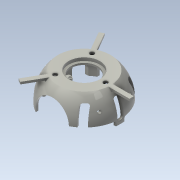
# Autodesk Inventor part: RobotHoedje
Saved by Autodesk Inventor 2020.3 (Build 243373000, 373)
## iProperties
Created: 2020-10-22
Part Number: RobotHoedje
Material: Acetal Resin, Black
Document SubType Name: Modeling
Designer: Britt
Density: 1.425 g/cm^3
Appearance: Smooth - Ivory
Author: Britt
Autodesk Inventor part; units mm, degrees
ref_plane "YZ Plane" through (0, 0, 0) normal (1, 0, 0) x (0, 1, 0)
ref_plane "XZ Plane" through (0, 0, 0) normal (0, 1, 0) x (-1, 0, 0)
ref_plane "XY Plane" through (0, 0, 0) normal (0, 0, 1) x (1, 0, 0)
sketch "Sketch1" plane through (0, 0, 0) normal (0, 1, 0) x (-1, 0, 0)
  circle A0 centre (0, 0) radius 81.5
  line L0 (0, 81.5) -> (0, 79.5)
  line L1 (0, 79.5) -> (17.9444, 79.5)
  line L2 (0, 79.5) -> (-17.9444, 79.5)
  dimension "d0" = 163
  dimension "d13" = 2
  constraints: 6 end point, 3 point on circle, 1 centre point, 1 coincident, 1 perpendicular, 1 point on line, 1 vertical
  measures "d0" diameter of A0
  measures "d13" distance of L0.start L0.end
extrude "Extrusion1" add sketch "Sketch1" along normal blind 90 contours A0 L2 L1
fillet "Fillet1" radius 80 1 edges at (0, 90, -81.5)
shell "Shell1" thickness 5 removed faces 1 at (-16.0199, 0, 6.9823)
sketch "Sketch3" plane through (-17.9444, 0, 79.5) normal (0, 0, 1) x (1, 0, 0)
  line L0 (17.9444, 0) -> (17.9444, 10)
  circle A0 centre (17.9444, 10) radius 37.5
  line L1 (-19.5556, 10) -> (-19.5556, 0)
  line L2 (55.4444, 10) -> (55.4444, 0)
  line L3 (99.4444, 0) -> (-63.5556, 0) projected
  line L4 (55.4444, 0) -> (-19.5556, 0)
  line L5 (0, 0) -> (35.8887, 0) projected
  dimension "d14" = 10
  dimension "d15" = 75
  constraints: 8 end point, 3 vertical, 2 point on circle, 1 centre point, 1 coincident, 1 collinear, 1 point on line, 1 tangent
  measures "d14" distance of L0.start L0.end
  measures "d15" diameter of A0
extrude "Extrusion3" cut sketch "Sketch3" against normal through all both and the other way through all contours A0 L3 | L2 L3 A0 | A0 L3 L1 picked at (4.1693, 13.1062)
sketch "Sketch5" plane through (0, 90, 0) normal (0, 1, 0) x (1, 0, 0)
  circle A0 centre (0, 0) radius 1.5 projected
  circle A1 centre (0, 0) radius 35.5
  dimension "d24" = 71
  constraints: 1 centre point, 1 coincident
  measures "d24" diameter of A1
extrude "Extrusion5" cut sketch "Sketch5" against normal through all
ref_plane "Work Plane3" through (0, 78, 0) normal (0, 1, 0) x (1, 0, 0)
sketch "Sketch6" plane through (0, 78, 0) normal (0, 1, 0) x (1, 0, 0)
  line L0 (-10, -40.5) -> (10, -40.5)
  circle A0 centre (0, 0) radius 35.5 projected
  line L1 (10, -30.5) -> (-10, -40.5) construction
  line L2 (-10, -30.5) -> (10, -40.5) construction
  line L3 (10, 40.5) -> (-10, 40.5)
  line L4 (10, 40.5) -> (-10, 30.5) construction
  line L5 (-10, 40.5) -> (10, 30.5) construction
  line L6 (-40.5, -10) -> (-40.5, 10)
  line L7 (-30.5, -10) -> (-40.5, 10) construction
  line L8 (-40.5, -10) -> (-30.5, 10) construction
  line L9 (40.5, 10) -> (40.5, -10)
  line L10 (30.5, 10) -> (40.5, -10) construction
  line L11 (40.5, 10) -> (30.5, -10) construction
  circle A1 centre (0, 0) radius 40.5
  point P0 (0, -35.5)
  point P1 (0, 35.5)
  point P2 (-35.5, 0)
  point P3 (35.5, 0)
  dimension "d28" = 20
  dimension "d29" = 10
  dimension "d30" = 20
  dimension "d31" = 10
  dimension "d32" = 10
  dimension "d33" = 20
  dimension "d34" = 10
  dimension "d35" = 20
  constraints: 24 end point, 8 midpoint, 4 point on circle, 1 centre point, 1 coincident, 1 horizontal
  measures "d28" distance of L0.end L0.start
  measures "d29" distance of L2.start L0.start
  measures "d30" distance of L5.end L4.end
  measures "d31" distance of L4.end L3.end
  measures "d32" distance of L6.end L8.end
  measures "d33" distance of L6.start L6.end
  measures "d34" distance of L9.end L11.end
  measures "d35" distance of L9.start L9.end
extrude "Extrusion6" add sketch "Sketch6" against normal blind 20
sketch "Sketch7" plane through (0, 58, 0) normal (0, -1, 0) x (1, 0, 0)
  circle A0 centre (0, 0) radius 1.5 projected
  circle A1 centre (0, 0) radius 38.5714
  circle A2 centre (0, 0) radius 30
  dimension "d38" = 60
  constraints: 2 centre point, 2 coincident
  measures "d38" diameter of A2
extrude "Extrusion7" add sketch "Sketch7" along normal blind 4 contours A1
sketch "Sketch8" plane through (0, 0, 0) normal (0, -1, 0) x (1, 0, 0)
  arc A0 (76.2643, 6) -> (38.7342, 65.969) centre (0, 0) ccw projected
  line L0 (61.5, 6) -> (76.2643, 6) projected
  line L1 (76.097, 6) -> (81.2788, 6)
  arc A1 (41.2658, -70.2807) -> (41.2658, 70.2807) centre (0, 0) ccw projected
  line L2 (76.2643, -6) -> (61.5, -6) projected
  line L3 (76.097, -6) -> (81.2788, -6)
  line L4 (39.2915, 69.117) -> (34.9018, 73.1705)
  line L5 (34.9018, 73.1705) -> (33.5102, 67.8706)
  line L6 (33.5102, 67.8706) -> (38.7342, 65.969)
  line L7 (41.2658, -70.2807) -> (36.538, -72.9193)
  line L8 (36.538, -72.9193) -> (34.4671, -67.6441)
  arc A2 (38.7342, -65.969) -> (76.2643, -6) centre (0, 0) ccw projected
  line L9 (34.4671, -67.6441) -> (38.7342, -65.969)
  line L10 (76.097, 6) -> (61.5, 6)
  line L11 (33.5102, 67.8706) -> (61.5, 6)
  line L12 (61.5, -6) -> (34.4671, -67.6441)
  line L13 (81.2788, -6) -> (84.4133, -6)
  line L14 (84.4133, -6) -> (69.6893, -61.2083)
  line L15 (69.6893, -61.2083) -> (36.538, -72.9193)
  line L16 (81.2788, 6) -> (84.4133, 6)
  line L17 (84.4133, 6) -> (69.5528, 69.3789)
  line L18 (69.5528, 69.3789) -> (34.9018, 73.1705)
  line L19 (76.097, 6) -> (75.9085, 9.4949)
  arc A3 (-37.5, 66.6783) -> (-37.5, -66.6783) centre (0, 0) ccw projected
  line L20 (75.9085, 9.4949) -> (83.5938, 9.4949)
  line L21 (75.9085, 9.4949) -> (59.9189, 9.4949)
  line L22 (76.097, -6) -> (75.9085, -9.4949)
  line L23 (75.9085, -9.4949) -> (83.4812, -9.4949)
  line L24 (75.9085, -9.4949) -> (59.8849, -9.4949)
  point P0 (41.2658, 70.0874)
  point P1 (41.2658, 70.2807)
  point P2 (59.9674, -9.4949)
  dimension "d153" = 3.5
  dimension "d154" = 3.5
  constraints: 46 end point, 6 point on line, 4 horizontal, 3 point on circle, 1 collinear, 1 parallel, 1 perpendicular
  measures "d153" distance of L1.start L19.end
  measures "d154" distance of L3.start L22.end
extrude "Extrusion23" cut sketch "Sketch8" against normal blind 10 contours L21 L11 L6 A0 | A0 L6 L5 L18 L17 L20 | L7 L8 L9 A2 L23 A1 | A1 L23 L14 L15 L7 | A2 L9 L12 L24
sketch "Sketch9" plane through (0, 85, 0) normal (0, -1, 0) x (1, 0, 0)
  circle A0 centre (0, 0) radius 38.5714 projected
  line L0 (0, 38.5714) -> (-15, 38.5714)
  line L1 (-15, 38.5714) -> (-15, 68.5714)
  line L2 (-15, 68.5714) -> (0, 68.5714)
  line L3 (0, 68.5714) -> (0, 38.5714)
  line L4 (0, 38.5714) -> (15, 38.5714)
  line L5 (15, 38.5714) -> (15, 68.5714)
  line L6 (15, 68.5714) -> (0, 68.5714)
  line L7 (0, 68.5714) -> (0, 38.5714)
  arc A1 (-40.5, 0) -> (-40.5, 0) centre (0, 0) ccw projected
  line L8 (0, -40.5) -> (-15, -40.5)
  line L9 (-15, -40.5) -> (-15, -70.5)
  line L10 (-15, -70.5) -> (0, -70.5)
  line L11 (0, -70.5) -> (0, -40.5)
  line L12 (0, -70.5) -> (15, -70.5)
  line L13 (15, -70.5) -> (15, -40.5)
  line L14 (15, -40.5) -> (0, -40.5)
  line L15 (0, -40.5) -> (0, -70.5)
  arc A2 (-40.5, 0) -> (-40.5, 0) centre (0, 0) ccw projected
  line L16 (40.5, 0) -> (70.5, 0)
  line L17 (70.5, 0) -> (70.5, 15)
  line L18 (70.5, 15) -> (40.5, 15)
  line L19 (40.5, 15) -> (40.5, 0)
  line L20 (70.5, 0) -> (40.5, 0)
  line L21 (40.5, 0) -> (40.5, -15)
  line L22 (40.5, -15) -> (70.5, -15)
  line L23 (70.5, -15) -> (70.5, 0)
  point P0 (0, 68.5714)
  dimension "d43" = 15
  dimension "d44" = 30
  dimension "d45" = 15
  dimension "d46" = 30
  dimension "d47" = 30
  dimension "d48" = 15
  dimension "d49" = 15
  constraints: 48 end point, 12 parallel, 6 horizontal, 6 perpendicular, 6 point on line, 2 point on circle, 2 other
  measures "d43" distance of L1.end L2.end
  measures "d44" distance of L0.end L1.end
  measures "d45" distance of L6.end L5.end
  measures "d46" distance of L9.end L8.end
  measures "d47" distance of L18.end L17.end
  measures "d48" distance of L17.end L16.end
  measures "d49" distance of L21.end L20.end
extrude "Extrusion9" cut sketch "Sketch9" along normal blind 20 contours L0 A1 L3 | L3 A1 L4 | L19 L18 L17 L16 | L16 L23 L22 L21 | L14 L13 L12 L11 | L11 L10 L9 L8 | L0 L1 L2 L3 A1 | L3 L6 L5 L4 A1
sketch "Sketch15" plane through (0, 0, 0) normal (0, -1, 0) x (1, 0, 0)
  arc A0 (-41.2658, 70.2807) -> (-41.2658, -70.2807) centre (0, 0) ccw projected
  line L0 (-81.5, 0) -> (-61.9, 0)
  line L1 (-61.9, 0) -> (-61.9, 30)
  line L2 (-61.9, 0) -> (-61.9, -30)
  line L3 (-61.9, -30) -> (-70.3722, -30) construction
  arc A1 (-38.7342, 65.969) -> (-38.7342, -65.969) centre (0, 0) ccw projected
  line L4 (-61.9, -25.75) -> (-70.3722, -25.75)
  line L5 (-70.3722, -34.25) -> (-61.9, -34.25)
  arc A2 (-61.9, -34.25) -> (-61.9, -25.75) centre (-61.9, -30) ccw
  arc A3 (-70.3722, -25.75) -> (-70.3722, -34.25) centre (-70.3722, -30) ccw
  line L6 (-61.9, 30) -> (-70.3722, 30) construction
  line L7 (-61.9, 34.25) -> (-70.3722, 34.25)
  line L8 (-70.3722, 25.75) -> (-61.9, 25.75)
  arc A4 (-61.9, 25.75) -> (-61.9, 34.25) centre (-61.9, 30) ccw
  arc A5 (-70.3722, 34.25) -> (-70.3722, 25.75) centre (-70.3722, 30) ccw
  point P0 (-66.1361, -30)
  point P1 (-66.1361, 30)
  point P2 (-71.9296, -26.0456)
  point P3 (-68.4046, -34.25)
  dimension "d84" = 19.6
  dimension "d85" = 30
  dimension "d86" = 30
  dimension "d87" = 8.5
  dimension "d88" = 8.5
  constraints: 22 end point, 11 point on circle, 8 tangent, 4 centre point, 3 parallel, 2 horizontal, 2 midpoint, 1 perpendicular, 1 vertical
  measures "d84" distance of L0.start L0.end
  measures "d85" distance of L0.end L1.end
  measures "d86" distance of L0.end L2.end
  measures "d87" diameter of A3
  measures "d88" diameter of A5
extrude "Extrusion13" add sketch "Sketch15" against normal blind 5 contours A5 L7 A1 | A1 L7 A4 L8 A5 | A3 L4 A2 L5 A1
sketch "Sketch16" plane through (0, 5, 0) normal (0, 1, 0) x (1, 0, 0)
  arc A0 (-61.9, 25.75) -> (-61.9, 34.25) centre (-61.9, 30) ccw projected
  arc A1 (-61.9, -34.25) -> (-61.9, -25.75) centre (-61.9, -30) ccw projected
  point P0 (0, 0)
  constraints: 2 coincident
hole "Hole4" at (-61.9, 5, -30) at (-61.9, 5, 30) direction (0, -1, 0) diameter 3.2 end through all
sketch "Sketch17" plane through (0, 5, 0) normal (0, 1, 0) x (1, 0, 0)
  circle A0 centre (-61.9, 30) radius 1.6 projected
  line L0 (-61.9, 33.2043) -> (-59.125, 31.6021)
  line L1 (-59.125, 31.6021) -> (-59.125, 28.3979)
  line L2 (-59.125, 28.3979) -> (-61.9, 26.7957)
  line L3 (-61.9, 26.7957) -> (-64.675, 28.3979)
  line L4 (-64.675, 28.3979) -> (-64.675, 31.6021)
  line L5 (-64.675, 31.6021) -> (-61.9, 33.2043)
  circle A1 centre (-61.9, -30) radius 1.6 projected
  line L6 (-64.7188, -28.4763) -> (-61.9899, -26.797)
  line L7 (-61.9899, -26.797) -> (-59.171, -28.3207)
  line L8 (-59.171, -28.3207) -> (-59.0812, -31.5237)
  line L9 (-59.0812, -31.5237) -> (-61.8101, -33.203)
  line L10 (-61.8101, -33.203) -> (-64.629, -31.6793)
  line L11 (-64.629, -31.6793) -> (-64.7188, -28.4763)
  point P0 (0, 0)
  dimension "d98" = 5.55
  dimension "d99" = 5.55
  constraints: 24 end point, 2 coincident, 26 other
  measures "d98" distance between parallel lines of L4 L1
  measures "d99" distance between parallel lines of L11 L8
extrude "Extrusion14" cut sketch "Sketch17" against normal blind 3
sketch "Sketch18" plane through (0, 78, 0) normal (0, 1, 0) x (1, 0, 0)
  circle A0 centre (0, 0) radius 1.5
  constraints: 1 centre point, 1 coincident
extrude "Extrusion15" cut sketch "Sketch18" along normal through all
sketch "Sketch19" plane through (0, 65, 0) normal (0, 1, 0) x (1, 0, 0)
  circle A0 centre (0, 0) radius 59.5948
  constraints: 1 centre point, 1 coincident
extrude "Extrusion16" cut sketch "Sketch19" along normal through all
sketch "Sketch20" plane through (0, 65, 0) normal (0, 1, 0) x (1, 0, 0)
  circle A0 centre (0, 0) radius 35.5
  circle A1 centre (0, 0) radius 59.5948
  constraints: 2 centre point, 2 coincident
extrude "Extrusion17" add sketch "Sketch20" against normal blind 5
sketch "Sketch21" plane through (0, 65, 0) normal (0, 1, 0) x (1, 0, 0)
  circle A0 centre (0, 0) radius 57.4017 projected
  line L0 (57.4017, 0) -> (107.4017, 0)
  line L1 (107.4017, 0) -> (107.4017, -5)
  line L2 (107.4017, -5) -> (57.4017, -5)
  line L3 (57.4017, -5) -> (57.4017, 0)
  line L4 (107.4017, -5) -> (57.4017, -5)
  line L5 (57.4017, -5) -> (57.4017, 5)
  line L6 (57.4017, 5) -> (107.4017, 5)
  line L7 (107.4017, 5) -> (107.4017, -5)
  line L8 (-28.7008, 49.7113) -> (-53.7008, 93.0126)
  line L9 (-28.7008, -49.7113) -> (-53.7008, -93.0126)
  line L10 (-28.7008, -49.7113) -> (-24.3707, -52.2113)
  line L11 (-28.7008, -49.7113) -> (-23.7008, -49.7113) construction
  line L12 (-24.3707, -52.2113) -> (-49.3707, -95.5126)
  line L13 (-49.3707, -95.5126) -> (-58.031, -90.5126)
  line L14 (-58.031, -90.5126) -> (-33.031, -47.2113)
  line L15 (-33.031, -47.2113) -> (-24.3707, -52.2113)
  line L16 (-28.7008, 49.7113) -> (-24.3707, 52.2113)
  line L17 (-28.7008, 49.7113) -> (-23.7008, 49.7113) construction
  line L18 (-24.3707, 52.2113) -> (-49.3707, 95.5126)
  line L19 (-49.3707, 95.5126) -> (-58.031, 90.5126)
  line L20 (-58.031, 90.5126) -> (-33.031, 47.2113)
  line L21 (-33.031, 47.2113) -> (-24.3707, 52.2113)
  dimension "d108" = 50
  dimension "d109" = 5
  dimension "d110" = 10
  dimension "d111" = 50
  dimension "d112" = 50
  dimension "d113" = 5
  dimension "d114" = 30
  dimension "d115" = 50
  dimension "d116" = 90
  dimension "d117" = 10
  dimension "d118" = 50
  dimension "d119" = 5
  dimension "d120" = 30
  dimension "d121" = 10
  dimension "d122" = 50
  constraints: 44 end point, 7 perpendicular, 4 horizontal, 4 parallel, 3 point on line, 2 equal length, 1 coincident, 1 horizontal alignment, 6 other
  measures "d108" distance of L1.end L2.end
  measures "d109" distance of L0.end L1.end
  measures "d110" distance of L4.end L5.end
  measures "d111" distance of L8.start L8.end
  measures "d112" distance of L9.start L9.end
  measures "d113" distance of L9.start L10.end
  measures "d114" angle of L10 L11
  measures "d115" distance of L10.end L12.end
  measures "d116" angle of L10 L12
  measures "d117" distance of L12.end L13.end
  measures "d118" distance of L13.end L14.end
  measures "d119" distance of L8.start L16.end
  measures "d120" angle of L17 L16
  measures "d121" distance of L18.end L19.end
  measures "d122" distance of L19.end L20.end
extrude "Extrusion18" add sketch "Sketch21" against normal blind 5 contours L10 L12 L13 L9 | L9 L13 L14 L15 | L21 L20 L19 L8 | L8 L19 L18 L16 | L5 L6 L7 L0 | L0 L1 L2 L3
fillet "Fillet3" radius 2 3 edges at (-31.975, 60, 55.3823) (-31.975, 60, -55.3823) (63.95, 60, 0)
sketch "Sketch22" plane through (0, 0, 0) normal (0, -1, 0) x (1, 0, 0)
  line L0 (-49.3707, 95.5126) -> (-58.031, 90.5126) projected
  line L1 (-49.3707, -95.5126) -> (-58.031, -90.5126) projected
  arc A0 (-68.4046, -34.25) -> (-38.7342, -65.969) centre (0, 0) ccw projected
  line L2 (-49.3707, -58.4361) -> (-49.3707, -38.4361)
  line L3 (-49.3707, -38.4361) -> (-74.4178, -38.4361)
  line L4 (-74.4178, -38.4361) -> (-74.4178, -58.4361)
  line L5 (-74.4178, -58.4361) -> (-49.3707, -58.4361)
  line L6 (-49.3707, -58.4361) -> (-39.5116, -58.4361)
  line L7 (-38.2296, -56.2156) -> (-58.031, -90.5126) projected
  line L8 (-49.3707, -38.4361) -> (-39.5116, -58.4361)
  arc A1 (-38.7342, 65.969) -> (-68.4046, 34.25) centre (0, 0) ccw projected
  line L9 (-48.1303, 59.462) -> (-48.1303, 39.462)
  line L10 (-48.1303, 39.462) -> (-74.4178, 39.462)
  line L11 (-74.4178, 39.462) -> (-74.4178, 59.462)
  line L12 (-74.4178, 59.462) -> (-48.1303, 59.462)
  line L13 (-48.1303, 59.462) -> (-40.1039, 59.462)
  line L14 (-34.0224, 48.9286) -> (-58.031, 90.5126) projected
  line L15 (-48.1303, 39.462) -> (-40.1039, 59.462)
  dimension "d126" = 20
  dimension "d139" = 20
  constraints: 24 end point, 4 parallel, 2 horizontal, 2 perpendicular, 2 point on circle, 2 point on line, 1 vertical
  measures "d126" distance of L2.start L2.end
  measures "d139" distance of L9.start L9.end
extrude "Extrusion19" cut sketch "Sketch22" against normal blind 25 contours L3 L2 A0 | A0 L5 L4 L3 | L2 L8 L6 | L9 L10 A1 | L13 L15 L9 | A1 L10 L11 L12
fillet "Fillet4" radius 10 4 edges at (-50.8722, 25, -58.4361) (-67.3194, 25, -38.4361) (-49.6618, 25, 59.462) (-66.7221, 25, 39.462)
sketch "Sketch26" plane through (0, 65, 0) normal (0, 1, 0) x (1, 0, 0)
  line L0 (48.2507, 0) -> (-24.1254, -41.7863)
  line L1 (-24.1254, -41.7863) -> (-24.1254, 41.7863)
  line L2 (-24.1254, 41.7863) -> (48.2507, 0)
  circle A0 centre (-24.1254, 41.7863) radius 5
  circle A1 centre (-24.1254, -41.7863) radius 5
  circle A2 centre (48.2507, 0) radius 5
  point P0 (0, 0)
  dimension "d140" = 10
  dimension "d141" = 10
  dimension "d142" = 10
  constraints: 6 end point, 3 centre point, 3 coincident, 7 other
  measures "d140" diameter of A0
  measures "d141" diameter of A1
  measures "d142" diameter of A2
extrude "Extrusion21" cut sketch "Sketch26" against normal blind 10 contours L2 A2 L0 | L0 A2 L2 | A1 L1 L0 | L0 L1 A1 | A0 L1 L2 | L2 L1 A0
sketch "Sketch27" plane through (107.4017, 65, 5) normal (1, 0, 0) x (0, 0, -1)
  line L0 (5, -65) -> (5, 0)
  line L1 (40.5, 0) -> (-30.5, 0) projected
  line L2 (5, -65) -> (5, -30)
  line L3 (5, -30) -> (-30, -30)
  line L4 (5, -30) -> (40, -30) construction
  line L5 (-30, -30) -> (40, -30)
  circle A0 centre (-30, -30) radius 3
  circle A1 centre (40, -30) radius 3
  dimension "d145" = 35
  dimension "d146" = 35
  dimension "d147" = 180
  dimension "d148" = 70
  dimension "d149" = 6
  dimension "d150" = 6
  constraints: 10 end point, 2 centre point, 2 coincident, 2 horizontal, 2 point on line, 1 collinear, 1 midpoint
  measures "d145" distance of L0.start L2.end
  measures "d146" distance of L2.end L3.end
  measures "d147" angle of L3 L4
  measures "d148" distance of L3.end L5.end
  measures "d149" diameter of A0
  measures "d150" diameter of A1
extrude "Extrusion22" cut sketch "Sketch27" against normal through all
sketch "Sketch29" plane through (0, 10, 0) normal (0, -1, 0) x (1, 0, 0)
  arc A0 (80.945, -9.4949) -> (80.945, 9.4949) centre (0, 0) ccw projected
  line L0 (81.5, 0) -> (81.5, -6)
  line L1 (81.5, 0) -> (87.5, 0) construction
  line L2 (81.5, -6) -> (60.1489, -6)
  line L3 (60.1489, -6) -> (60.1489, 6)
  line L4 (81.5, 0) -> (81.5, 6)
  line L5 (81.5, 6) -> (60.1489, 6)
  dimension "d157" = 6
  dimension "d158" = 90
  dimension "d159" = 12
  constraints: 12 end point, 4 perpendicular, 2 tangent, 2 vertical, 1 horizontal, 1 point on circle
  measures "d157" distance of L0.start L0.end
  measures "d158" angle of L0 L1
  measures "d159" distance of L2.end L3.end
extrude "Extrusion24" cut sketch "Sketch29" along normal blind 2 and the other way blind 40
fillet "Fillet6" radius 5 4 edges at (78.4267, 10, 9.4949) (78.4267, 10, -9.4949) (78.7716, 8, 6) (78.7716, 8, -6)
fillet "Fillet7" radius 5 2 edges at (67.5962, 50, 6) (67.5962, 50, -6)
sketch "Sketch30" plane through (0, 10, 0) normal (0, -1, 0) x (1, 0, 0)
  line L0 (81.4939, 0) -> (81.4939, -65)
  line L1 (81.4939, -65) -> (46.4939, -65)
  line L2 (0, 70.0988) -> (56, 70.0988)
  line L3 (56, 70.0988) -> (56, 60.0988)
  line L4 (56, 60.0988) -> (41.339, 28.6582)
  line L5 (56, 60.0988) -> (90.6909, 60.0988) construction
  line L6 (41.339, 28.6582) -> (34.0885, 32.0391)
  line L7 (34.0885, 32.0391) -> (48.5895, 25.2773)
  line L8 (48.5895, 25.2773) -> (65.1092, 60.704)
  line L9 (65.1092, 60.704) -> (50.6083, 67.4659)
  line L10 (50.6083, 67.4659) -> (34.0885, 32.0391)
  line L11 (-0.2382, -70.5392) -> (55.7618, -70.5392)
  line L12 (55.7618, -70.5392) -> (55.7618, -60.5392)
  line L13 (55.7618, -60.5392) -> (39.9851, -26.706)
  line L14 (55.7618, -60.5392) -> (93.0926, -60.5392) construction
  line L15 (39.9851, -26.706) -> (47.2356, -23.3251)
  line L16 (47.2356, -23.3251) -> (32.7346, -30.087)
  line L17 (32.7346, -30.087) -> (51.5978, -70.5392)
  line L18 (51.5978, -70.5392) -> (66.0988, -63.7773)
  line L19 (66.0988, -63.7773) -> (47.2356, -23.3251)
  point P0 (0, 0)
  point P1 (49.0149, -65)
  point P2 (66.2336, -65)
  point P3 (55.7618, -65)
  point P4 (63.4767, -65)
  point P5 (55.7618, -68.5975)
  dimension "d166" = 65
  dimension "d167" = 35
  dimension "d168" = 56
  dimension "d169" = 10
  dimension "d170" = 115
  dimension "d171" = 8
  dimension "d172" = 16
  dimension "d173" = 90
  dimension "d174" = 90
  dimension "d175" = 56
  dimension "d176" = 10
  dimension "d177" = 115
  dimension "d178" = 8
  dimension "d179" = 90
  dimension "d180" = 90
  dimension "d181" = 16
  dimension "d182" = 90
  constraints: 40 end point, 7 perpendicular, 4 horizontal, 3 point on line, 2 equal length, 2 vertical
  measures "d166" distance of L0.start L0.end
  measures "d167" distance of L0.end L1.end
  measures "d168" distance of L2.start L2.end
  measures "d169" distance of L2.end L3.end
  measures "d170" angle of L4 L5
  measures "d171" distance of L4.end L6.end
  measures "d172" distance of L6.end L7.end
  measures "d173" angle of L8 L7
  measures "d174" angle of L9 L8
  measures "d175" distance of L11.start L11.end
  measures "d176" distance of L11.end L12.end
  measures "d177" angle of L14 L13
  measures "d178" distance of L13.end L15.end
  measures "d179" angle of L13 L15
  measures "d180" angle of L17 L16
  measures "d181" distance of L17.end L18.end
  measures "d182" angle of L18 L17
extrude "Extrusion25" cut sketch "Sketch30" against normal blind 40 contours L1 L12 L13 L15 L19 L18 | L1 L17 L16 L13 L12 | L9 L8 L7 L4 L3 | L3 L4 L6 L10 L9
fillet "Fillet8" radius 5 4 edges at (43.1329, 50, -52.3861) (54.9274, 50, -39.8203) (55.1963, 50, 39.4457) (43.4527, 50, 52.1208)
sketch "Sketch31" plane through (0, 58, 0) normal (0, -1, 0) x (1, 0, 0)
  circle A0 centre (0, 0) radius 40.5
  circle A1 centre (0, 0) radius 38.5714 projected
  circle A2 centre (0, 0) radius 38.5714
  constraints: 2 centre point, 2 coincident
extrude "Extrusion26" add sketch "Sketch31" along normal blind 4
body "Solid1"
